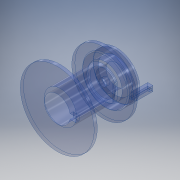
# Autodesk Inventor part: 电机帽
Saved by Autodesk Inventor 2018 (Build 220112000, 112)
## iProperties
Created: 2020-11-22
Part Number: 电机帽
Material: 水
Document SubType Name: Modeling
Designer: OHHHHHHHHHH
Density: 0.9983 g/cm^3
Appearance: 热带地区蓝色
Author: OHHHHHHHHHH
## iProperties of the stored document 电机帽_3D 打印.ipt
Created: 2020-11-30
Part Number: 电机帽_3D 打印
Material: 常规
Document SubType Name: Modeling
Designer: OHHHHHHHHHH
Density: 1 g/cm^3
Appearance: 默认
Author: OHHHHHHHHHH
Autodesk Inventor part; units mm, degrees
ref_plane "YZ Plane" through (0, 0, 0) normal (1, 0, 0) x (0, 1, 0)
ref_plane "XZ Plane" through (0, 0, 0) normal (0, 1, 0) x (-1, 0, 0)
ref_plane "XY Plane" through (0, 0, 0) normal (0, 0, 1) x (1, 0, 0)
sketch "草图1" plane through (0, 0, 0) normal (0, 1, 0) x (-1, 0, 0)
  circle A0 centre (0, 0) radius 35.5
  dimension "d0" = 71
  constraints: 1 centre point, 1 coincident
  measures "d0" diameter of A0
extrude "拉伸1" add sketch "草图1" along normal blind 3
sketch "草图2" plane through (0, 3, 0) normal (0, 1, 0) x (1, 0, 0)
  circle A0 centre (0, 0) radius 15.5
  circle A1 centre (0, 0) radius 12.5
  dimension "d3" = 31
  dimension "d4" = 25
  constraints: 2 centre point, 2 coincident
  measures "d3" diameter of A0
  measures "d4" diameter of A1
extrude "拉伸2" add sketch "草图2" along normal blind 41
sketch "草图3" plane through (0, 44, 0) normal (0, 1, 0) x (1, 0, 0)
  circle A0 centre (0, 0) radius 30
  dimension "d7" = 60
  constraints: 1 centre point, 1 coincident
  measures "d7" diameter of A0
extrude "拉伸3" add sketch "草图3" along normal blind 3
sketch "草图4" plane through (0, 0, 0) normal (0, -1, 0) x (1, 0, 0)
  circle A0 centre (0, 0) radius 12.5 projected
extrude "拉伸4" cut sketch "草图4" against normal blind 3
sketch "草图5" plane through (0, 47, 0) normal (0, 1, 0) x (1, 0, 0)
  circle A0 centre (0, 0) radius 12.5 projected
  circle A1 centre (0, 0) radius 3.5
  dimension "d12" = 7
  constraints: 1 centre point, 1 coincident
  measures "d12" diameter of A1
extrude "拉伸5" cut sketch "草图5" against normal blind 5 contours A1
sketch "草图6" plane through (0, 47, 0) normal (0, 1, 0) x (1, 0, 0)
  circle A0 centre (0, 0) radius 10
  circle A1 centre (0, 0) radius 22.5
  dimension "d15" = 20
  dimension "d16" = 45
  constraints: 2 centre point, 2 coincident
  measures "d15" diameter of A0
  measures "d16" diameter of A1
extrude "拉伸6" add sketch "草图6" along normal blind 10
sketch "草图7" plane through (0, 47, 0) normal (0, 1, 0) x (1, 0, 0)
  circle A0 centre (0, 0) radius 3.5 projected
  line L0 (3.5, 3.5) -> (48.5, 3.5)
  line L1 (48.5, 3.5) -> (48.5, -3.5)
  line L2 (48.5, -3.5) -> (3.5, -3.5)
  line L3 (3.5, -3.5) -> (3.5, 3.5)
  dimension "d19" = 45
  dimension "d20" = 7
  constraints: 8 end point, 2 parallel, 2 tangent, 1 horizontal, 1 perpendicular
  measures "d19" distance of L0.start L0.end
  measures "d20" distance of L0.end L1.end
extrude "拉伸7" [suppressed]
sketch "草图8" plane through (0, 47, 0) normal (0, 1, 0) x (1, 0, 0)
  circle A0 centre (44.1819, 0) radius 2.5
  point P0 (0, 0)
  dimension "d23" = 5
  constraints: 1 centre point
  measures "d23" diameter of A0
extrude "拉伸8" [suppressed]
pattern_circular "环形阵列1" [suppressed]
sketch "草图9" plane through (0, 47, 0) normal (0, 1, 0) x (1, 0, 0)
  line L0 (24, -2.5) -> (29, -2.5)
  line L1 (29, -2.5) -> (29, 2.5)
  line L2 (29, 2.5) -> (24, 2.5)
  line L3 (24, 2.5) -> (24, -2.5)
  line L4 (-49.7, 0) -> (49.7, 0) projected
  point P0 (0, 0)
  dimension "d32" = 5
  dimension "d33" = 5
  dimension "d34" = 24
  constraints: 8 end point, 2 parallel, 1 horizontal, 1 perpendicular, 1 other
  measures "d32" distance of L2.end L0.start
  measures "d33" distance of L0.start L0.end
  measures "d34" distance from line of L3 point (0, 0)
extrude "拉伸9" add sketch "草图9" along normal blind 16
sketch "草图10" plane through (0, 44, 0) normal (0, -1, 0) x (1, 0, 0)
  line L0 (13.5, 10) -> (26.5, 10)
  line L1 (26.5, 10) -> (26.5, -12)
  line L2 (26.5, -12) -> (13.5, -12)
  line L3 (13.5, -12) -> (13.5, 10)
  point P0 (0, 0)
  dimension "d36" = 10
  dimension "d38" = 22
  dimension "d40" = 13
  dimension "d41" = 13.5
  constraints: 8 end point, 2 parallel, 1 horizontal, 1 perpendicular
  measures "d36" distance from line of L0 point (0, 0)
  measures "d38" distance of L0.end L1.end
  measures "d40" distance of L0.start L0.end
  measures "d41" distance from line of point (0, 0) L3
extrude "拉伸10" cut sketch "草图10" along normal blind 4
sketch "草图11" plane through (0, 44, 0) normal (0, -1, 0) x (1, 0, 0)
  circle A0 centre (0, 0) radius 12.5 projected
  line L0 (24, 2.5) -> (29, 2.5) projected
  line L1 (29, 2.5) -> (29, -2.5) projected
  line L2 (29, -2.5) -> (24, -2.5) projected
  line L3 (24, -2.5) -> (24, 2.5) projected
  line L4 (27.5, -1) -> (27.5, 1)
  line L5 (27.5, 1) -> (25.5, 1)
  line L6 (25.5, 1) -> (25.5, -1)
  line L7 (25.5, -1) -> (27.5, -1)
  dimension "d44" = 1.5
  constraints: 8 end point, 3 other
  measures "d44" distance between parallel lines of L1 L4
extrude "拉伸11" cut sketch "草图11" against normal blind 17.5 contours L7 L6 L5 L4
sketch "草图12" plane through (29, 47, 2.5) normal (1, 0, 0) x (0, 0, -1)
  line L0 (1.5, 14.5) -> (3.5, 14.5) projected
  line L1 (3.5, -3) -> (3.5, 14.5) projected
  line L2 (1.5, 14.5) -> (3.5, 14.5)
  line L3 (3.5, 14.5) -> (3.5, 12.5)
  line L4 (3.5, 12.5) -> (1.5, 12.5)
  line L5 (1.5, 12.5) -> (1.5, 14.5)
  point P0 (2.5, -47)
  dimension "d47" = 2
  constraints: 8 end point, 2 parallel, 1 horizontal, 1 perpendicular, 1 point on line
  measures "d47" distance between parallel lines of L0 L4
extrude "拉伸12" cut sketch "草图12" against normal blind 2
sketch "草图13" plane through (0, 0, 0) normal (0, -1, 0) x (1, 0, 0)
  line L0 (24, -2.5) -> (29, -2.5) projected
  line L1 (9, 2.3127) -> (18, 2.3127)
  line L2 (18, 2.3127) -> (18, -2.5)
  line L3 (18, -2.5) -> (9, -2.5)
  line L4 (9, -2.5) -> (9, 2.3127)
  point P0 (0, 0)
  dimension "d52" = 9
  dimension "d53" = 9
  constraints: 8 end point, 2 parallel, 1 horizontal, 1 perpendicular, 1 point on line
  measures "d52" distance from line of L4 point (0, 0)
  measures "d53" distance between parallel lines of L4 L2
extrude "拉伸13" cut sketch "草图13" against normal blind 3
ref_plane "工作平面2" through (0, 56, 0) normal (0, 1, 0) x (1, 0, 0)
sketch "草图14" plane through (0, 57, 0) normal (0, 1, 0) x (1, 0, 0)
  circle A0 centre (0, 0) radius 10 projected
  circle A1 centre (0, 0) radius 22.5 projected
  arc A2 (13.5, -7.6158) -> (13.5, 7.6158) centre (0, 0) ccw projected
  arc A3 (13.5, 7.6158) -> (13.5, -7.6158) centre (0, 0) ccw projected
  circle A4 centre (0, 0) radius 21.5
  arc A5 (14.371, -8.1071) -> (14.371, 8.1071) centre (0, 0) ccw
  arc A6 (14.371, 8.1071) -> (14.371, -8.1071) centre (0, 0) ccw
  dimension "d56" = 1
  constraints: 4 point on circle, 3 centre point, 1 other
  measures "d56" radial gap between concentric circles of A3 A6
sketch "草图15" plane through (0, 56, 0) normal (0, 1, 0) x (1, 0, 0)
  circle A0 centre (0, 0) radius 10
  circle A1 centre (0, 0) radius 22.5
  arc A2 (13.5, -7.6158) -> (13.5, 7.6158) centre (0, 0) ccw
  arc A3 (13.5, 7.6158) -> (13.5, -7.6158) centre (0, 0) ccw
  circle A4 centre (0, 0) radius 21.5
  arc A5 (14.371, -8.1071) -> (14.371, 8.1071) centre (0, 0) ccw
  arc A6 (14.371, 8.1071) -> (14.371, -8.1071) centre (0, 0) ccw
  dimension "d58" = 1
  constraints: 8 point on circle, 7 centre point, 1 other
  measures "d58" radial gap between concentric circles of A3 A6
extrude "拉伸14" cut sketch "草图15" against normal blind 10 contours A4
